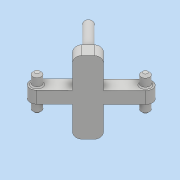
# Autodesk Inventor part: corps
Saved by Autodesk Inventor 2017 (Build 210142000, 142)
## iProperties
Created: 2017-12-31
Part Number: corps
Material: Generic
Document SubType Name: Modeling
Designer: Aegir
Density: 1 g/cm^3
Appearance: Default
Author: Aegir
Autodesk Inventor part; units mm, degrees
ref_plane "YZ Plane" through (0, 0, 0) normal (1, 0, 0) x (0, 1, 0)
ref_plane "XZ Plane" through (0, 0, 0) normal (0, 1, 0) x (-1, 0, 0)
ref_plane "XY Plane" through (0, 0, 0) normal (0, 0, 1) x (1, 0, 0)
sketch "Esquisse1" plane through (0, 0, 0) normal (0, 0, 1) x (1, 0, 0)
  circle A0 centre (-5.1667, 0) radius 4 projected
  circle A1 centre (-5.1667, 0) radius 4
  circle A2 centre (-54.8562, -49.0632) radius 4 projected
  circle A3 centre (-54.8562, -49.0632) radius 4
  point P0 (0, 0)
  constraints: 2 centre point, 2 coincident, 2 concentric
extrude "Extrusion1" add sketch "Esquisse1" against normal blind 10
sketch "Esquisse2" plane through (-5.1667, 0, 0) normal (0, 0, 1) x (1, 0, 0)
  circle A0 centre (0, 0) radius 4
  circle A1 centre (0, 0) radius 6.3333
  circle A2 centre (0, 0) radius 4.3
  arc A3 (4.2132, -4.7287) -> (-4.4886, 4.4681) centre (0, 0) ccw
  line L0 (-115.082, -98.1727) -> (98.3913, 112.6096)
  line L1 (-115.082, -98.1727) -> (98.3913, 112.6096)
  line L2 (-115.082, -98.1727) -> (98.3913, 112.6096)
  circle A4 centre (-49.6895, -49.0632) radius 4
  circle A5 centre (-49.6895, -49.0632) radius 6.3333
  circle A6 centre (-49.6895, -49.0632) radius 4.3
  line L3 (4.6759, -4.2717) -> (-45.2392, -53.5693)
  line L4 (-4.4107, 4.545) -> (-54.1394, -44.5565)
  arc A7 (4.2132, -4.7287) -> (-4.4886, 4.4681) centre (0, 0) ccw
  arc A8 (-54.1394, -44.5565) -> (-45.2392, -53.5693) centre (-49.6895, -49.0632) ccw
  point P0 (5.1667, 0)
extrude "Extrusion2" add sketch "Esquisse2" along normal blind 5.5 contours A0 | A1 L3 | A1 L3 A5 L4 | A5 | A2 | A4 | A6 picked at (5.5499, -0.8587)
mirror "Symétrie1" about plane through (-54.8562, -49.0632, 5.5) normal (0, 0, 1) of "Extrusion1", "Extrusion2"
sketch "Esquisse4" plane through (-0.4908, -4.2717, 0) normal (0.7027, -0.7115, 0) x (0.7115, 0.7027, 0)
  line L0 (-70.1545, 0) -> (-70.1545, 11) projected
  line L1 (-70.1545, 0) -> (-70.1553, 0) projected
  line L2 (-70.1553, 0) -> (-70.1553, 11) projected
  line L3 (-70.1545, 11) -> (-70.1553, 11) projected
  line L4 (-70.1553, 0) -> (0, 0) projected
  line L5 (0, 0) -> (0, 11) projected
  line L6 (-70.1553, 11) -> (0, 11) projected
  line L7 (-70.1553, 0) -> (-70.1553, 11) projected
  line L8 (0, 0) -> (-0.2696, 0) projected
  line L9 (-0.2696, 0) -> (-0.2696, 11) projected
  line L10 (0, 11) -> (-0.2696, 11) projected
  line L11 (0, 0) -> (0, 11) projected
  line L12 (-41.2971, -27.5) -> (-33.2971, -27.5)
  line L13 (-27.2971, -21.5) -> (-27.2971, 32.5)
  line L14 (-33.2971, 38.5) -> (-41.2971, 38.5)
  line L15 (-47.2971, 32.5) -> (-47.2971, -21.5)
  line L16 (-151.1905, -5.5) -> (148.8095, -5.5) projected
  line L17 (148.8095, -5.5) -> (148.8095, 16.5) projected
  line L18 (-151.1905, 16.5) -> (148.8095, 16.5) projected
  line L19 (-151.1905, -5.5) -> (-151.1905, 16.5) projected
  arc A0 (-47.2971, -21.5) -> (-41.2971, -27.5) centre (-41.2971, -21.5) ccw
  arc A1 (-33.2971, -27.5) -> (-27.2971, -21.5) centre (-33.2971, -21.5) ccw
  arc A2 (-27.2971, 32.5) -> (-33.2971, 38.5) centre (-33.2971, 32.5) ccw
  arc A3 (-41.2971, 38.5) -> (-47.2971, 32.5) centre (-41.2971, 32.5) ccw
  point P0 (3.3509, 0)
  point P1 (-47.2971, -27.5)
  point P2 (-27.2971, -27.5)
  point P3 (-47.2971, 38.5)
  dimension "d4" = 20
  dimension "d5" = 55.7149
  dimension "d6" = 20
  dimension "d7" = 22.8574
  dimension "d8" = 66
  dimension "d9" = 22
  dimension "d10" = 6
  constraints: 8 end point, 8 point on circle, 8 tangent, 6 point on line, 4 centre point, 3 equal radius, 2 parallel, 1 horizontal, 1 perpendicular
  measures "d4" distance between parallel lines of L13 L15
  measures "d6" distance of point (-47.297, -27.5) point (-27.297, -27.5)
  measures "d7" distance from line of L0 point (-47.297, -27.5)
  measures "d8" distance of point (-47.297, 38.5) point (-47.297, -27.5)
  measures "d9" distance between parallel lines of L16 L12
  measures "d10" radius of A0
extrude "Extrusion3" add sketch "Esquisse4" against normal blind 12 contours L15 L6 L13 L4 | L4 L13 L16 L15 | L15 L18 L13 L6 | L16 L13 A1 L12 A0 L15 | L15 A3 L14 A2 L13 L18
sketch "Esquisse5" plane through (-8.9231, 4.2662, 0) normal (-0.7027, 0.7115, 0) x (0.7115, 0.7027, 0)
  circle A0 centre (-37.2971, -27.5) radius 4
  ellipse E0 centre (-35.2029, -27.5) end of major axis (-35.2029, -31.5) minor radius 4 projected
  line L0 (-47.2971, -11) -> (-47.2971, -32.5) projected
  line L1 (-151.1905, 5.5) -> (148.8095, 5.5) projected
  line L2 (148.8095, 5.5) -> (148.8095, -16.5) projected
  line L3 (-151.1905, -16.5) -> (148.8095, -16.5) projected
  line L4 (-151.1905, 5.5) -> (-151.1905, -16.5) projected
  circle A1 centre (-37.2971, 16.5) radius 4
  line L5 (-47.2971, 21.5) -> (-47.2971, 0) projected
  point P0 (3.3509, 0)
  dimension "d13" = 4
  dimension "d14" = 8
  dimension "d15" = 10
  dimension "d16" = 11
  dimension "d17" = 8
  dimension "d18" = 10
  dimension "d19" = 11
  constraints: 2 centre point, 1 other
  measures "d14" diameter of A0
  measures "d15" distance from line of L0 A0.centre
  measures "d16" distance from line of L3 A0.centre
  measures "d17" diameter of A1
  measures "d18" distance from line of L5 A1.centre
  measures "d19" distance from line of L1 A1.centre
extrude "Extrusion4" add sketch "Esquisse5" along normal blind 40 contours A0 E0 | E0 A0 | A1 picked at (-37.2152, -27.4202) picked at (-40.5742, -27.6143)
chamfer "Chanfrein1" distance 2 angle 45 6 edges at (-66.4134, 3.7068, -16.5) (-66.4134, 3.7068, 27.5) (-9.1667, 0, 21) (-9.1667, 0, -10) (-58.8562, -49.0632, -10) (-58.8562, -49.0632, 21)
sketch "Esquisse6" plane through (-63.5674, 6.5176, -16.5) normal (-0.7027, 0.7115, 0) x (0.7115, 0.7027, 0)
  circle A0 centre (0, -44) radius 4 projected
  circle A1 centre (0, 0) radius 4 projected
  circle A2 centre (0, -44) radius 4
  circle A3 centre (0, -44) radius 3.9
  circle A4 centre (0, 0) radius 4
  circle A5 centre (0, 0) radius 3.9
  point P0 (40.648, -16.5)
  dimension "d25" = 8
  dimension "d26" = 7.8
  dimension "d27" = 7.8
  constraints: 4 centre point, 4 coincident, 2 concentric
  measures "d25" diameter of A0
  measures "d26" diameter of A3
  measures "d27" diameter of A5
extrude "Extrusion5" cut sketch "Esquisse6" against normal blind 40
sketch "Esquisse7" plane through (-5.1667, 0, -10) normal (0, 0, -1) x (-1, 0, 0)
  circle A0 centre (0, 0) radius 4 projected
  circle A1 centre (49.6895, -49.0632) radius 4 projected
  circle A2 centre (0, 0) radius 4
  circle A3 centre (0, 0) radius 3.9
  circle A4 centre (49.6895, -49.0632) radius 4
  circle A5 centre (49.6895, -49.0632) radius 3.9
  point P0 (-5.1667, 0)
  dimension "d30" = 8
  dimension "d31" = 7.8
  dimension "d32" = 7.8
  constraints: 4 centre point, 4 coincident, 2 concentric
  measures "d30" diameter of A0
  measures "d31" diameter of A3
  measures "d32" diameter of A5
extrude "Extrusion6" cut sketch "Esquisse7" against normal up to surface (10 mm away)
sketch "Esquisse8" plane through (-54.8562, -49.0632, 21) normal (0, 0, 1) x (1, 0, 0)
  circle A0 centre (0, 0) radius 4 projected
  circle A1 centre (49.6895, 49.0632) radius 4 projected
  circle A2 centre (0, 0) radius 4
  circle A3 centre (0, 0) radius 3.9
  circle A4 centre (49.6895, 49.0632) radius 4
  circle A5 centre (49.6895, 49.0632) radius 3.9
  point P0 (54.8562, 49.0632)
  dimension "d35" = 8
  dimension "d36" = 7.8
  dimension "d37" = 7.8
  constraints: 4 centre point, 4 coincident, 2 concentric
  measures "d35" diameter of A1
  measures "d36" diameter of A5
  measures "d37" diameter of A3
extrude "Extrusion7" cut sketch "Esquisse8" against normal up to surface (10 mm away)
chamfer "Chanfrein2" distance 2 angle 45 2 edges at (-38.2346, -24.6827, -16.5) (-38.2346, -24.6827, 27.5)
chamfer "Chanfrein3" distance 1 angle 45 4 edges at (-9.0667, 0, 11) (-1.2667, 0, 0) (-50.9562, -49.0632, 0) (-58.7562, -49.0632, 11)
equation "\"d26\" = d27"
equation "\"d32\" = d31"
equation "\"d37\" = d36"
